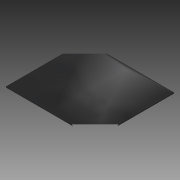
# Autodesk Inventor part: ElectronicsLowerPanel
Saved by Autodesk Inventor 2015 SP1 (Build 190203100, 203)
## iProperties
Category: Panel
Created: 2015-01-14
Part Number: ElectronicsLowerPanel
Material: ABS Plastic
Document SubType Name: Modeling
Designer: Jack
Density: 1.06 g/cm^3
Appearance: Smooth - Dark Gray
Mass: 818.214 g
Surface Area: 3929.9 cm^2
Volume: 771.9 cm^3
Vendor: Tap Plastics
Catalog Web Link: N/A
Author: Jack
Title: Electronics Lower Panel
Autodesk Inventor part; units mm, degrees
ref_plane "YZ Plane" through (0, 0, 0) normal (1, 0, 0) x (0, 1, 0)
ref_plane "XZ Plane" through (0, 0, 0) normal (0, 1, 0) x (-1, 0, 0)
ref_plane "XY Plane" through (0, 0, 0) normal (0, 0, 1) x (1, 0, 0)
sketch "Sketch1" plane through (0, 0, 0) normal (0, 0, 1) x (1, 0, 0)
  line L0 (0, 0) -> (430, 0)
  line L1 (430, 0) -> (430, 380)
  line L2 (430, 380) -> (0, 380)
  line L3 (0, 380) -> (0, 0)
  dimension "d0" = 430
  dimension "d1" = 380
  constraints: 8 end point, 2 parallel, 1 horizontal, 1 perpendicular
  measures "d0" distance of L2.end L1.end
  measures "d1" distance of L1.end L0.end
extrude "Extrusion1" add sketch "Sketch1" along normal blind 4.7625
sketch "Sketch2" plane through (0, 0, 4.7625) normal (0, 0, 1) x (1, 0, 0)
  line L0 (0, 0) -> (430, 0) projected
  line L1 (430, 0) -> (430, 380) projected
  line L2 (430, 380) -> (0, 380) projected
  line L3 (0, 380) -> (0, 0) projected
  point P0 (16, 364)
  point P1 (215, 364)
  point P2 (16, 16)
  point P3 (215, 16)
  point P4 (414, 16)
  point P5 (414, 364)
  dimension "d8" = 215
  dimension "d17" = 16
  dimension "d18" = 16
  dimension "d19" = 16
  dimension "d20" = 16
  constraints: 5 horizontal alignment, 3 vertical alignment
  measures "d8" distance from line of L1 point (215, 16)
  measures "d17" distance from line of L2 point (215, 364)
  measures "d18" distance from line of L3 point (16, 364)
  measures "d19" distance from line of L1 point (414, 364)
  measures "d20" distance from line of L0 point (215, 16)
hole "Hole1" at (16, 364, 4.7625) at (215, 364, 4.7625) at (16, 16, 4.7625) at (215, 16, 4.7625) at (414, 16, 4.7625) at (414, 364, 4.7625) direction (0, 0, -1) diameter 3 end through all
body "Solid1"
